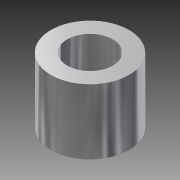
# Autodesk Inventor part: 25312-14
Saved by Autodesk Inventor 2014 (Build 180170000, 170)
## iProperties
Category: stocked
Created: 2013-07-17
Part Number: 25312-14
Material: Aluminum 6061
Document SubType Name: Modeling
Designer: Edward
Density: 2.71 g/cm^3
Appearance: Aluminum - Polished
Catalog Web Link: aluminumspacers.com
Vendor: aluminumspacers.com
Stock Number: AS38-12-20
Description: 3/8" x 5/16" x #12 bore, aluminum spacer
Project: Shapeoko
User Status: F
Mass: 1.01242 g
Surface Area: 4.70511 cm^2
Volume: 0.373586 cm^3
Authority: ALUMINUMSPACERS.COM, 8-2-13
d0: 5.560 mm
d1: 9.530 mm
d2: 7.940 mm
d3: 0.00 deg
Author: Edward
Subject: Spacers
Comments: Fusion
Autodesk Inventor part; units mm, degrees
ref_plane "YZ Plane" through (0, 0, 0) normal (1, 0, 0) x (0, 1, 0)
ref_plane "XZ Plane" through (0, 0, 0) normal (0, 1, 0) x (-1, 0, 0)
ref_plane "XY Plane" through (0, 0, 0) normal (0, 0, 1) x (1, 0, 0)
sketch "Sketch1" plane through (0, 0, 0) normal (0, 0, 1) x (1, 0, 0)
  circle A0 centre (0, 0) radius 2.78
  circle A1 centre (0, 0) radius 4.765
  dimension "d0" = 5.56
  dimension "d1" = 9.53
  constraints: 2 centre point, 2 coincident
  measures "d0" diameter of A0
  measures "d1" diameter of A1
extrude "Extrusion1" add sketch "Sketch1" along normal blind 7.94
body "Solid1"
